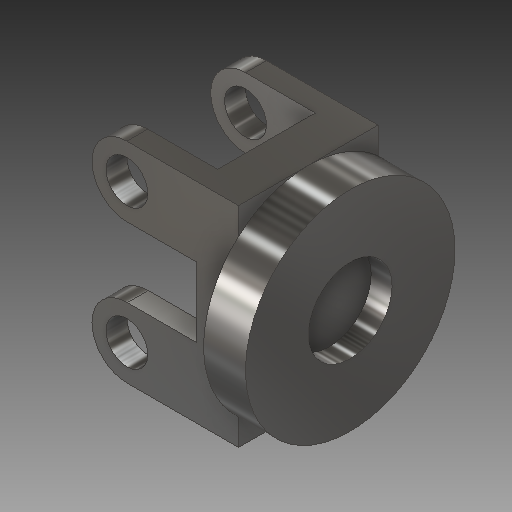
# Autodesk Inventor part: Wrist
Saved by Autodesk Inventor 2019 (Build 230136000, 136)
## iProperties
Created: 2018-12-28
Part Number: Wrist
Material: 钢，高强度，低合金
Document SubType Name: Modeling
Designer: JianQiao Hu
Density: 7.85 g/cm^3
Appearance: 钢 - 抛光
Author: JianQiao Hu
Autodesk Inventor part; units mm, degrees
ref_plane "YZ Plane" through (0, 0, 0) normal (1, 0, 0) x (0, 1, 0)
ref_plane "XZ Plane" through (0, 0, 0) normal (0, 1, 0) x (-1, 0, 0)
ref_plane "XY Plane" through (0, 0, 0) normal (0, 0, 1) x (1, 0, 0)
sketch "草图1" plane through (0, 0, 0) normal (0, 0, 1) x (1, 0, 0)
  line L0 (-40, 25) -> (40, 25)
  line L1 (40, 25) -> (40, -25)
  line L2 (40, -25) -> (-40, -25)
  line L3 (-40, 25) -> (40, -25) construction
  line L4 (40, 25) -> (-40, -25) construction
  arc A0 (-40, 25) -> (-40, -25) centre (-40, 0) ccw
  circle A1 centre (-40, 0) radius 15
  line L5 (-39.6714, -125) -> (39.6714, -125)
  line L6 (39.6714, -125) -> (39.6714, -75)
  line L7 (39.6714, -75) -> (-39.6714, -75)
  line L8 (-39.6714, -125) -> (39.6714, -75) construction
  line L9 (39.6714, -125) -> (-39.6714, -75) construction
  arc A2 (-39.6714, -75) -> (-39.6714, -125) centre (-40, -100) ccw
  circle A3 centre (-40, -100) radius 15
  point P0 (0, 0)
  point P1 (0, -100)
  dimension "d0" = 50
  dimension "d3" = 30
  dimension "d11" = 50
  dimension "d12" = 30
  dimension "d13" = 100
  dimension "d14" = 0
  dimension "d15" = 25
  dimension "d16" = 80
  constraints: 20 end point, 4 centre point, 4 midpoint, 4 point on circle, 2 coincident, 2 horizontal, 2 parallel, 2 perpendicular
  measures "d0" distance of L0.end L1.end
  measures "d3" diameter of A1
  measures "d11" distance of L5.end L6.end
  measures "d12" diameter of A3
  measures "d13" distance of A1.centre A3.centre
  measures "d14" horizontal distance of A3.centre A1.centre
  measures "d15" radius of A0
  measures "d16" distance from line of L1 A1.centre
extrude "拉伸1" add sketch "草图1" along normal mid plane 100
sketch "草图2" plane through (-40, 25, 50) normal (0, 1, 0) x (1, 0, 0)
  line L0 (40, 50) -> (0, 50)
  line L1 (0, 100) -> (0, 0) projected
  line L2 (50, 85) -> (-98.1355, 85)
  line L3 (-98.1355, 85) -> (-98.1355, 15)
  line L4 (-98.1355, 15) -> (50, 15)
  line L5 (50, 15) -> (50, 85)
  line L6 (50, 85) -> (-98.1355, 15) construction
  line L7 (-98.1355, 85) -> (50, 15) construction
  line L8 (80, 0) -> (80, 100) projected
  point P0 (-24.0677, 50)
  dimension "d4" = 30
  dimension "d5" = 70
  constraints: 14 end point, 3 midpoint, 2 parallel, 1 horizontal, 1 perpendicular, 1 point on line
  measures "d4" distance between parallel lines of L8 L5
  measures "d5" distance of L2.end L3.end
extrude "拉伸2" cut sketch "草图2" against normal through all
sketch "草图3" plane through (40, -25, 50) normal (1, 0, 0) x (0, 0, -1)
  line L0 (100, 50) -> (0, 50) projected
  line L1 (0, 50) -> (100, 50)
  line L2 (100, 50) -> (100, -100)
  line L3 (100, -100) -> (0, -100)
  line L4 (0, -100) -> (0, 50)
  point P0 (50, 25)
  point P1 (15, 50)
  dimension "d8" = 150
  constraints: 8 end point, 2 parallel, 1 horizontal, 1 perpendicular
  measures "d8" distance of L0.start L2.end
extrude "拉伸3" add sketch "草图3" against normal blind 30
sketch "草图4" plane through (40, -125, 50) normal (1, 0, 0) x (0, 0, -1)
  line L0 (100, 100) -> (100, 50) projected
  line L1 (100, 75) -> (0, 75)
  line L2 (0, 0) -> (0, 150) projected
  line L3 (15, 0) -> (85, 0) projected
  line L4 (50, 0) -> (50, 150)
  line L5 (0, 150) -> (100, 150) projected
  circle A0 centre (50, 75) radius 75
  point P0 (50, 125)
  constraints: 5 midpoint, 4 end point, 1 vertical alignment, 2 other
extrude "拉伸4" add sketch "草图4" along normal blind 30 contours L4 A0 L2 L1 | L4 A0 | L1 L2 A0 L4 | L2 A0
sketch "草图5" plane through (70, -50, 0) normal (1, 0, 0) x (0, 0, -1)
  circle A0 centre (0, 0) radius 30
  point P0 (0, 50)
  dimension "d19" = 60
  constraints: 1 centre point
  measures "d19" diameter of A0
extrude "拉伸5" cut sketch "草图5" against normal blind 15
